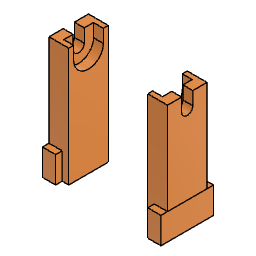
WaterMillPart v5 (Autodesk Fusion 360 design; units mm, degrees)
Autodesk Fusion 360 part; units mm, degrees
note: some values were not read from the file. Chosen so that the rebuilt part matches the saved one: which face or edge a step refers to.
sketch "Sketch1" plane through (0, 0, 0) normal (0, 0, 1) x (1, 0, 0)
  line L0 (45, 100) -> (-45, 100)
  line L1 (-45, 100) -> (-45, -100)
  line L2 (-45, -100) -> (45, -100)
  line L3 (45, -100) -> (45, 100)
  line L4 (45, 100) -> (-45, -100) construction
  line L5 (-45, 100) -> (45, -100) construction
  dimension "d1" = 200
  dimension "d2" = 90
  constraint horizontal L0
  constraint perpendicular L0 L1
  constraint parallel L0 L2
  constraint parallel L1 L3
  constraint coincident L4 origin
  constraint coincident L5 origin
  measures "d1" distance of L0.end L1.end
  measures "d2" distance of L1.end L2.end
extrude "Extrude1" add sketch "Sketch1" along normal blind 10 makes body 1
sketch "Sketch2" plane through (0, 0, 10) normal (0, 0, 1) x (-1, 0, 0)
  line L0 (-45, 100) -> (-45, -100)
  line L1 (-45, -100) -> (45, -100)
  line L2 (45, -100) -> (45, 100)
  line L3 (45, 100) -> (-45, 100)
  line L4 (-35, -90) -> (35, -90)
  line L5 (35, 90) -> (-35, 90)
  line L6 (-35, -90) -> (35, 90) construction
  line L7 (35, -90) -> (-35, 90) construction
  line L8 (0, -100) -> (0, 100) construction
  line L9 (45, 0) -> (-45, 0) construction
  line L10 (35, -15) -> (30, -15)
  line L11 (30, -15) -> (30, 0)
  line L12 (35, -90) -> (35, -15)
  line L13 (35, 15) -> (35, 90)
  line L14 (30, 15) -> (30, 0)
  line L15 (35, 15) -> (30, 15)
  line L16 (-35, -15) -> (-30, -15)
  line L17 (-30, -15) -> (-30, 0)
  line L18 (-30, 15) -> (-30, 0)
  line L19 (-35, 15) -> (-30, 15)
  line L20 (-35, 90) -> (-35, 15)
  line L21 (-35, -15) -> (-35, -90)
  dimension "d5" = 10
  dimension "d6" = 10
  dimension "d7" = 5
  dimension "d8" = 15
  constraint horizontal L4
  constraint perpendicular L4 L12
  constraint parallel L4 L5
  constraint parallel L12 L20
  constraint coincident L6 origin
  constraint coincident L7 origin
  constraint midpoint L1 L8.start
  constraint midpoint L3 L8.end
  constraint midpoint L2 L9.start
  constraint midpoint L0 L9.end
  constraint perpendicular L10 L12
  constraint coincident L9 L11.end
  constraint perpendicular L9 L11
  constraint collinear L12 L13
  constraint symmetric L9 L10.start L13.start
  constraint symmetric L9 L10.end L14.start
  constraint symmetric L9 L11.end L14.end
  constraint symmetric L8 L10.start L16.start
  constraint symmetric L8 L10.end L16.end
  constraint symmetric L8 L11.end L17.end
  constraint symmetric L8 L14.start L18.start
  constraint symmetric L8 L13.start L19.start
  constraint collinear L20 L21
  measures "d5" distance of L1 L4
  measures "d6" distance of L2 L12
  measures "d7" distance of L10.start L10.end
  measures "d8" distance of L10.end L11.end
extrude "Extrude2" add sketch "Sketch2" along normal blind 50 bodies 1
sketch "Sketch3" plane through (0, 0, 60) normal (0, 0, 1) x (-1, 0, 0)
  line L0 (-35, -15) -> (-30, -15)
  line L1 (-30, -15) -> (-30, 15)
  line L2 (-30, 15) -> (-35, 15)
  line L3 (-35, 15) -> (-35, 90)
  line L4 (-35, 90) -> (35, 90)
  line L5 (35, 90) -> (35, 15)
  line L6 (35, 15) -> (30, 15)
  line L7 (30, 15) -> (30, -15)
  line L8 (30, -15) -> (35, -15)
  line L9 (35, -15) -> (35, -90)
  line L10 (35, -90) -> (-35, -90)
  line L11 (-35, -90) -> (-35, -15)
  line L12 (45, 100) -> (-45, 100)
  line L13 (-45, 100) -> (-45, -100)
  line L14 (-45, -100) -> (45, -100)
  line L15 (45, -100) -> (45, 100)
  line L16 (0, -100) -> (0, 100) construction
  line L17 (45, 0) -> (-45, 0) construction
  line L18 (30, -15) -> (45, -15)
  line L19 (30, -15) -> (30, 15)
  line L20 (45, 15) -> (30, 15)
  line L21 (45, -15) -> (45, 15)
  line L22 (-30, -15) -> (-35, -15)
  line L23 (-30, -15) -> (-30, 15)
  line L24 (-45, -15) -> (-45, 15)
  line L25 (-30, -15) -> (-45, -15)
  line L26 (-30, 15) -> (-30, -15)
  line L27 (-45, 15) -> (-30, 15)
  line L28 (-35, 15) -> (-30, 15)
  point P0 (-45, 0)
  constraint midpoint L14 L16.start
  constraint midpoint L12 L16.end
  constraint midpoint L15 L17.start
  constraint midpoint L13 P0
  constraint coincident L7.end L8.start
  constraint coincident L15 L18.end
  constraint perpendicular L15 L18
  constraint coincident L6.end L7.start
  constraint coincident L15 L20.start
  constraint perpendicular L7 L20
  constraint symmetric L5.end L16 L2.end
  constraint symmetric L6.end L16 L1.end
  constraint symmetric L7.end L16 L0.end
  constraint symmetric L8.end L16 L0.start
  constraint symmetric L16 L17.start P0
  constraint symmetric L16 L7.end L0.end
  constraint symmetric L16 L18.end L24.start
  constraint symmetric L16 L6.end L1.end
  constraint symmetric L16 L20.start L24.end
extrude "Extrude3" add sketch "Sketch3" along normal blind 80 contours L0 L1 L2 L13 L22 L23 L24 L25 L26 L27 L28 | L6 L7 L8 L15 L18 L19 L20 L21 bodies 1
sketch "Sketch4" plane through (-30, 0, 0) normal (1, 0, 0) x (0, 1, 0)
  line L0 (-15, 10) -> (15, 10)
  line L1 (15, 10) -> (15, 140)
  line L2 (15, 140) -> (-15, 140)
  line L3 (-15, 140) -> (-15, 10)
  line L4 (-11.25, 160) -> (-11.25, 120)
  arc A0 (-11.25, 120) -> (11.25, 120) centre (0, 120) ccw
  line L5 (11.25, 120) -> (11.25, 160)
  arc A1 (11.25, 160) -> (-11.25, 160) centre (0, 160) ccw
  line L6 (0, 160) -> (0, 120) construction
  line L7 (-15, 60) -> (15, 60)
  point P0 (0, 140)
  dimension "d13" = 60
  dimension "d14" = 11.25
  constraint tangent L4 A0
  constraint tangent A0 L5
  constraint parallel L4 L5
  constraint tangent L5 A1
  constraint tangent L4 A1
  constraint perpendicular L2 L6
  constraint midpoint L2 P0
  constraint midpoint L6 P0
  measures "d13" distance of A0.centre L7
  measures "d14" radius of A0
extrude "Extrude4" cut sketch "Sketch4" against normal blind 7.5 contours L2 L4 A0 L5 bodies 1
sketch "Sketch5" plane through (-37.5, 0, 0) normal (1, 0, 0) x (0, 1, 0)
  line L0 (11.25, 120) -> (11.25, 140)
  line L1 (11.25, 140) -> (-11.25, 140)
  line L2 (-11.25, 140) -> (-11.25, 120)
  arc A0 (-11.25, 120) -> (11.25, 120) centre (0, 120) ccw
  line L3 (-4.25, 160) -> (-4.25, 120)
  arc A1 (-4.25, 120) -> (4.25, 120) centre (0, 120) ccw
  line L4 (4.25, 120) -> (4.25, 160)
  arc A2 (4.25, 160) -> (-4.25, 160) centre (0, 160) ccw
  line L5 (0, 160) -> (0, 120) construction
  point P0 (0, 140)
  dimension "d17" = 4.25
  constraint tangent L3 A1
  constraint tangent A1 L4
  constraint parallel L3 L4
  constraint tangent L4 A2
  constraint tangent L3 A2
  constraint coincident A0.centre A1.centre
  constraint perpendicular L1 L5
  constraint midpoint L1 P0
  constraint midpoint L5 P0
  measures "d17" radius of A1
extrude "Extrude5" cut sketch "Sketch5" against normal blind 7.5 contours L1 L3 A1 L4 bodies 1
mirror "Mirror1" about plane through (0, 0, 0) normal (1, 0, 0) of "Extrude4", "Extrude5"
sketch "Sketch6" plane through (0, 0, 60) normal (0, 0, 1) x (-1, 0, 0)
  line L0 (-45, 15) -> (-35, 15) construction
  line L1 (-35, 15) -> (-35, 90) construction
  line L2 (-35, 90) -> (35, 90) construction
  line L3 (35, 90) -> (35, 15) construction
  line L4 (35, 15) -> (45, 15) construction
  line L5 (45, 15) -> (45, 100) construction
  line L6 (45, 100) -> (-45, 100) construction
  line L7 (-45, 100) -> (-45, 15) construction
  line L8 (0, -100) -> (0, 100) construction
  line L9 (45, 0) -> (-45, 0) construction
  line L10 (45, 100) -> (35, 100)
  line L11 (35, 100) -> (35, 90)
  line L12 (35, 90) -> (45, 90)
  line L13 (45, 90) -> (45, 100)
  line L14 (-35, 100) -> (-35, 90)
  line L15 (-45, 90) -> (-45, 100)
  line L16 (-35, 90) -> (-45, 90)
  line L17 (-45, 100) -> (-35, 100)
  point P0 (-35, 90)
  point P1 (-45, 100)
  constraint midpoint L6 L8.end
  constraint perpendicular L6 L8
  constraint perpendicular L8 L9
  constraint horizontal L10
  constraint vertical L11
  constraint horizontal L12
  constraint vertical L13
  constraint coincident L2.end L3.start
  constraint coincident L5.end L6.start
  constraint symmetric L2.end L8 P0
  constraint symmetric L5.end L8 P1
  constraint symmetric L8 L5.end P1
  constraint symmetric L8 L10.end L14.start
  constraint symmetric L8 L2.end P0
  constraint symmetric L8 L12.end L15.start
move_face "OffsetFaces1" offset -10 1 faces at (-15, -100, 40) on bodies 1
move_face "OffsetFaces2" offset -70 1 faces at (-11.6667, -90, 3.3333) on bodies 1
move_face "OffsetFaces3" offset -20 1 faces at (-15, 100, 40) on bodies 1
move_face "OffsetFaces4" offset -60 1 faces at (11.6667, 80, 3.3333) on bodies 1
extrude "Extrude11" cut 4 faces at (42.5, -10.1667, 140) (42.5, 10.1667, 140) (-42.5, 10.1667, 140) (-42.5, -10.1667, 140) along direction (0, 0, -1) blind 10 on bodies 1 bodies 1
extrude "Extrude12" cut 1 faces at (10, -5, 10) along direction (0, 0, -1) blind 25 on bodies 1 bodies 1 makes body 2 at (-45, 5, 20)
extrude "Extrude13" cut 2 faces at (-41.6667, 5, 0) (41.6667, -5, 0) along direction (0, 0, 1) blind 40 on bodies 1 2 bodies 1 2
extrude "Extrude6" [suppressed]
sketch "Sketch7" plane through (0, 0, 160) normal (0, 0, 1) x (-1, 0, 0)
  line L0 (45, 90) -> (45, 100) construction
  line L1 (45, 100) -> (35, 100) construction
  line L2 (35, 100) -> (35, 90) construction
  line L3 (35, 90) -> (45, 90) construction
  line L4 (0, -100) -> (0, 100) construction
  line L5 (45, 0) -> (-45, 0) construction
  line L6 (45, 90) -> (35, 100) construction
  line L7 (35, 90) -> (45, 100) construction
  circle A0 centre (40, 95) radius 2.1625
  line L8 (-35, 90) -> (-45, 100) construction
  line L9 (-45, 100) -> (-35, 100) construction
  line L10 (-35, 100) -> (-35, 90) construction
  circle A1 centre (-40, 95) radius 2.1625
  line L11 (-35, 90) -> (-45, 90) construction
  line L12 (-45, 90) -> (-35, 100) construction
  line L13 (-45, 90) -> (-45, 100) construction
  dimension "d24" = 4.325
  constraint vertical L4
  constraint horizontal L5
  constraint coincident L0.start L3.end
  constraint coincident L1.end L2.start
  constraint coincident L2.end L3.start
  constraint coincident L0.end L1.start
  constraint midpoint L6 A0.centre
  constraint symmetric L0.start L4 L11.end
  constraint symmetric L0.end L4 L8.end
  constraint symmetric L1.end L4 L9.end
  constraint symmetric L2.end L4 L8.start
  constraint symmetric L4 L0.start L11.end
  constraint symmetric L4 L1.end L9.end
  constraint symmetric L4 L2.end L8.start
  constraint symmetric L4 L0.end L8.end
  constraint symmetric L4 A0 A1
  measures "d24" diameter of A0
extrude "Extrude7" [suppressed]
sketch "Sketch8" plane through (0, 0, 60) normal (0, 0, 1) x (-1, 0, 0)
  line L0 (45, 90) -> (35, 90) construction
  line L1 (35, 90) -> (35, 15) construction
  line L2 (35, 15) -> (45, 15) construction
  line L3 (45, 15) -> (45, 90) construction
  line L4 (0, 0) -> (0, 100) construction
  line L5 (40, 15) -> (40, 90) construction
  line L6 (45, 40) -> (35, 40)
  line L7 (35, 40) -> (35, 90)
  line L8 (35, 90) -> (45, 90)
  line L9 (45, 90) -> (45, 40)
  line L10 (-35, 90) -> (-45, 90)
  line L11 (-35, 40) -> (-35, 90)
  line L12 (-45, 90) -> (-45, 40)
  line L13 (-45, 40) -> (-35, 40)
  line L14 (-45, 90) -> (-35, 90) construction
  line L15 (45, 40) -> (35, 40) construction
  line L16 (-35, 40) -> (-45, 40) construction
  point P0 (-45, 52.5)
  point P1 (-40, 90)
  dimension "d33" = 50
  dimension "d34" = 10
  constraint coincident L4.start origin
  constraint perpendicular L4 L15
  constraint midpoint L2 L5.start
  constraint midpoint L0 L5.end
  constraint horizontal L6
  constraint vertical L7
  constraint horizontal L8
  constraint vertical L9
  constraint coincident L0.end L1.start
  constraint symmetric L0.start L4 L10.end
  constraint symmetric L0.end L4 L10.start
  constraint symmetric L6.start L4 L12.end
  constraint symmetric L4 L5.end P1
  constraint symmetric L4 L6.end L11.start
  constraint symmetric L4 L0.end L10.start
  constraint symmetric L4 L0.start L10.end
  constraint collinear L15 L16
  measures "d33" distance of L6.start L0.start
  measures "d34" distance of L6.start L6.end
extrude "Extrude8" [suppressed]
sketch "Sketch10" plane through (45, 0, 0) normal (1, 0, 0) x (0, 1, 0)
  line L0 (-100, 0) -> (100, 0)
  line L1 (100, 0) -> (100, 60)
  line L2 (100, 60) -> (15, 60)
  line L3 (15, 60) -> (-15, 60)
  line L4 (-15, 60) -> (-40, 60)
  line L5 (-40, 60) -> (-40, 135)
  line L6 (-40, 135) -> (-90, 135)
  line L7 (-90, 135) -> (-90, 160)
  line L8 (-90, 160) -> (-100, 160)
  line L9 (-100, 160) -> (-100, 0)
  line L10 (-90, 135) -> (-40, 60)
  line L11 (-40, 135) -> (-90, 135)
  line L12 (-40, 135) -> (-40, 60)
  constraint coincident L6.end L7.start
  constraint coincident L4.end L5.start
  constraint coincident L5.end L6.start
extrude "Extrude9" [suppressed]
sketch "Sketch11" plane through (-45, 0, 0) normal (-1, 0, 0) x (0, -1, 0)
  line L0 (90, 135) -> (40, 60)
  line L1 (40, 60) -> (15, 60)
  line L2 (15, 60) -> (-15, 60)
  line L3 (-15, 60) -> (-100, 60)
  line L4 (-100, 60) -> (-100, 0)
  line L5 (-100, 0) -> (100, 0)
  line L6 (100, 0) -> (100, 160)
  line L7 (100, 160) -> (90, 160)
  line L8 (90, 160) -> (90, 135)
  line L9 (-75, 50) -> (-75, 16)
  line L10 (-75, 50) -> (-66, 50)
  line L11 (-66, 50) -> (-63, 48)
  line L12 (-63, 48) -> (-63, 38)
  line L13 (-63, 38) -> (-67, 34)
  line L14 (-67, 34) -> (-71, 34)
  line L15 (-71, 34) -> (-71, 16)
  line L16 (-71, 16) -> (-75, 16)
  line L17 (-72, 46) -> (-72, 37)
  line L18 (-72, 37) -> (-69, 37)
  line L19 (-69, 37) -> (-66, 40)
  line L20 (-66, 40) -> (-66, 45)
  line L21 (-66, 45) -> (-66, 46)
  line L22 (-66, 46) -> (-72, 46)
  line L23 (-60, 16) -> (-50, 50)
  line L24 (-50, 50) -> (-46, 50)
  line L25 (-46, 50) -> (-38, 16)
  line L26 (-38, 16) -> (-41, 16)
  line L27 (-41, 16) -> (-44.5049, 30.8958)
  line L28 (-44.5049, 30.8958) -> (-53, 30.8958)
  line L29 (-53, 30.8958) -> (-57, 16)
  line L30 (-57, 16) -> (-60, 16)
  line L31 (-52.4349, 33) -> (-46, 33)
  line L32 (-46, 33) -> (-48, 44)
  line L33 (-48, 44) -> (-52.4349, 33)
  line L34 (-33, 50) -> (-33, 16)
  line L35 (-33, 16) -> (-30, 16)
  line L36 (-30, 16) -> (-30, 30)
  line L37 (-30, 30) -> (-24, 16)
  line L38 (-24, 16) -> (-22, 16)
  line L39 (-22, 16) -> (-28, 33)
  line L40 (-28, 33) -> (-21, 47)
  line L41 (-21, 47) -> (-23, 48)
  line L42 (-23, 48) -> (-30, 35)
  line L43 (-30, 35) -> (-30, 50)
  line L44 (-30, 50) -> (-33, 50)
  line L45 (-108, 38) -> (-105.6667, 41.5)
  dimension "d39" = 4.2065
  constraint vertical L9
  constraint perpendicular L9 L10
  constraint perpendicular L3 L12
  constraint perpendicular L9 L14
  constraint perpendicular L14 L15
  constraint perpendicular L9 L16
  constraint perpendicular L14 L17
  constraint perpendicular L17 L18
  constraint parallel L13 L19
  constraint parallel L17 L20
  constraint perpendicular L21 L22
  constraint perpendicular L9 L24
  constraint parallel L25 L27
  constraint parallel L24 L28
  constraint parallel L28 L30
  constraint parallel L30 L31
  constraint perpendicular L31 L34
  constraint perpendicular L34 L35
  constraint perpendicular L31 L36
  constraint perpendicular L36 L38
  constraint perpendicular L40 L41
  constraint parallel L36 L43
  constraint perpendicular L34 L44
  constraint perpendicular L11 L45
  measures "d39" distance of L45.start L45.end
extrude "Extrude10" [suppressed]
fillet "Fillet1" [suppressed]
